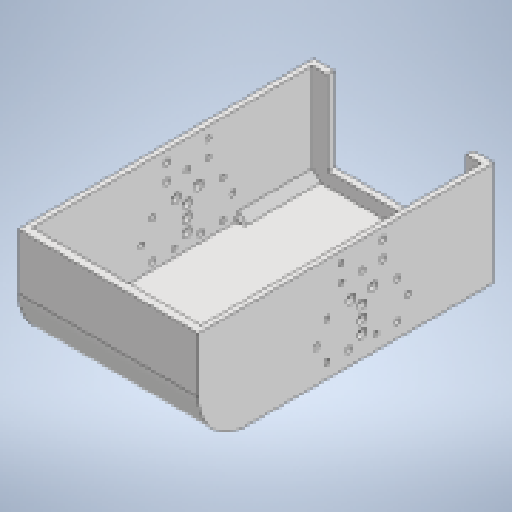
# Autodesk Inventor part: 车架
Saved by Autodesk Inventor 2025.1 (Build 291241000, 241)
## iProperties
Created: 2025-08-27
Part Number: 车架
Material: 常规
Document SubType Name: Modeling
Designer: Piw
Density: 1 g/cm^3
Appearance: 默认
Author: Piw
Autodesk Inventor part; units mm, degrees
ref_plane "YZ Plane" through (0, 0, 0) normal (1, 0, 0) x (0, 1, 0)
ref_plane "XZ Plane" through (0, 0, 0) normal (0, 1, 0) x (-1, 0, 0)
ref_plane "XY Plane" through (0, 0, 0) normal (0, 0, 1) x (1, 0, 0)
sketch "草图1" plane through (0, 0, 0) normal (0, 0, 1) x (1, 0, 0)
  line L0 (0, 5) -> (61, 5)
  line L1 (61, 5) -> (61, 75)
  line L2 (61, 75) -> (65, 75)
  line L3 (65, 75) -> (65, 0)
  line L4 (65, 0) -> (0, 0)
  line L5 (0, 34.2328) -> (0, -13.4923)
  line L6 (0, 5) -> (-61, 5)
  line L7 (-61, 5) -> (-61, 75)
  line L8 (-65, 75) -> (-65, 0)
  line L9 (-65, 0) -> (0, 0)
  line L10 (-61, 75) -> (-65, 75)
  dimension "d0" = 5
  dimension "d1" = 130
  dimension "d2" = 4
  dimension "d3" = 75
  constraints: 22 end point, 4 perpendicular, 4 symmetric about line, 2 vertical, 1 horizontal
  measures "d0" distance between parallel lines of L4 L0
  measures "d1" diameter of L3 L5
  measures "d2" distance between parallel lines of L3 L1
  measures "d3" distance between parallel lines of L4 L2
extrude "拉伸1" add sketch "草图1" along normal blind 138
sketch "草图2" plane through (65, 0, 0) normal (1, 0, 0) x (0, 0, -1)
  line L0 (-107.5, 24) -> (-72.5, 24) construction
  line L1 (0, 5) -> (-138, 5) projected
  circle A0 centre (-72.5, 24) radius 15.5 construction
  circle A1 centre (-107.5, 24) radius 15.5 construction
  circle A2 centre (-57, 24) radius 2.1
  circle A3 centre (-123, 24) radius 2.1
  line L2 (-138, 0) -> (-138, 75) projected
  circle A4 centre (-115.25, 10.5766) radius 2.1
  circle A5 centre (-99.75, 10.5766) radius 2.1
  circle A6 centre (-92, 24) radius 2.1
  circle A7 centre (-99.75, 37.4234) radius 2.1
  circle A8 centre (-115.25, 37.4234) radius 2.1
  circle A9 centre (-64.75, 37.4234) radius 2.1
  circle A10 centre (-80.25, 37.4234) radius 2.1
  circle A11 centre (-88, 24) radius 2.1
  circle A12 centre (-80.25, 10.5766) radius 2.1
  circle A13 centre (-64.75, 10.5766) radius 2.1
  point P0 (0, 0)
  dimension "d8" = 31
  dimension "d9" = 31
  dimension "d6" = 35
  dimension "d10" = 4.2
  dimension "d11" = 4.2
  dimension "d12" = 15
  dimension "d15" = 360
  dimension "d19" = 360
  dimension "d24" = 19
  constraints: 12 centre point, 2 coincident, 2 end point, 2 horizontal alignment, 2 point on line, 1 horizontal, 30 other
  measures "d6" distance of L0.start L0.end
  measures "d10" diameter of A2
  measures "d11" diameter of A3
  measures "d12" distance from line of L2 A3.centre
  measures "d24" distance between parallel lines of L1 L0
extrude "拉伸2" cut sketch "草图2" against normal blind 150 contours A2 | A3 | A4 | A5 | A8 | A9 | A12 | A13
sketch "草图3" plane through (65, 0, 0) normal (1, 0, 0) x (0, 0, -1)
  circle A0 centre (-90, 34) radius 3.25 projected
  circle A1 centre (-90, 25) radius 3.25 projected
  circle A2 centre (-90, 16) radius 3.25 projected
  circle A3 centre (-98, 41.2575) radius 3.25 projected
  circle A4 centre (-82, 41.2575) radius 3.25 projected
  point P0 (0, 0)
extrude "拉伸3" cut sketch "草图3" against normal blind 150
sketch "草图4" plane through (0, 0, 0) normal (0, 0, -1) x (-1, 0, 0)
  line L0 (-65, 0) -> (-65, 75) projected
  line L1 (65, 0) -> (-65, 0) projected
  line L2 (65, 75) -> (65, 0) projected
  line L3 (-65, 75) -> (-50, 75)
  line L4 (-50, 75) -> (-50, 15)
  line L5 (-50, 15) -> (50, 15)
  line L6 (50, 15) -> (50, 75)
  line L7 (50, 75) -> (65, 75)
  point P0 (0, 0)
  dimension "d27" = 15
  dimension "d28" = 15
  dimension "d29" = 15
  constraints: 10 end point, 4 perpendicular, 1 horizontal, 1 point on line
  measures "d27" distance between parallel lines of L1 L5
  measures "d28" distance between parallel lines of L2 L6
  measures "d29" distance between parallel lines of L4 L0
extrude "拉伸4" add sketch "草图4" along normal blind 5
sketch "草图5" plane through (0, 0, 0) normal (0, 0, 1) x (1, 0, 0)
  line L0 (61, 75) -> (61, 5) projected
  line L1 (50, 75) -> (61, 75) projected
  line L2 (50, 15) -> (50, 75) projected
  line L3 (-50, 15) -> (50, 15) projected
  line L4 (-50, 75) -> (-50, 15) projected
  line L5 (-61, 75) -> (-50, 75) projected
  line L6 (-61, 5) -> (-61, 75) projected
  line L7 (61, 5) -> (-61, 5) projected
  line L8 (61, 11) -> (55, 5)
  line L9 (0, 97.2027) -> (0, -45.2903)
  line L10 (-61, 11) -> (-55, 5)
  point P0 (0, 0)
  dimension "d32" = 45
  dimension "d33" = 6
  constraints: 6 end point, 2 point on line, 2 symmetric about line, 2 vertical
  measures "d32" angle of L0 L8
  measures "d33" horizontal distance of L8.end L8.start
extrude "拉伸5" add sketch "草图5" along normal blind 55 contours L0 L7 L8 | L7 L6 L10
chamfer "倒角1" distance 2 angle 45 2 edges at (58, 8, 55) (-58, 8, 55)
sketch "草图7" plane through (0, 0, 138) normal (0, 0, 1) x (1, 0, 0)
  line L0 (-65, 0) -> (65, 0) projected
  line L1 (65, 0) -> (65, 75) projected
  line L2 (65, 75) -> (61, 75) projected
  line L3 (61, 75) -> (61, 5) projected
  line L4 (61, 5) -> (-61, 5) projected
  line L5 (-61, 5) -> (-61, 75) projected
  line L6 (-61, 75) -> (-65, 75) projected
  line L7 (-65, 75) -> (-65, 0) projected
  point P0 (0, 0)
extrude "拉伸6" add sketch "草图7" along normal blind 25
sketch "草图13" plane through (-65, 0, -5) normal (-1, 0, 0) x (0, 0, 1)
  line L0 (80, 55) -> (110, 55) construction
  line L1 (110, 55) -> (110, 67) construction
  line L2 (110, 67) -> (80, 67) construction
  line L3 (80, 67) -> (80, 55) construction
  line L4 (80, 55) -> (110, 67) construction
  line L5 (110, 55) -> (80, 67) construction
  line L6 (0, 75) -> (168, 75) projected
  circle A0 centre (95, 34) radius 3.25 projected
  line L7 (95, 34) -> (95, 46.2012) construction
  circle A1 centre (80, 55) radius 2.1
  circle A2 centre (110, 55) radius 2.1
  circle A3 centre (95, 55) radius 2.1
  circle A4 centre (80, 67) radius 2.1
  circle A5 centre (110, 67) radius 2.1
  point P0 (5, 0)
  point P1 (95, 61)
  point P2 (233, 75)
  dimension "d62" = 8
  dimension "d63" = 30
  dimension "d64" = 20
  dimension "d65" = 4.2
  dimension "d66" = 4.2
  dimension "d67" = 4.2
  dimension "d68" = 4.2
  dimension "d69" = 4.2
  constraints: 14 end point, 5 centre point, 4 coincident, 3 midpoint, 2 parallel, 1 horizontal, 1 perpendicular, 1 point on line, 1 vertical
  measures "d62" distance between parallel lines of L6 L2
  measures "d63" distance between parallel lines of L1 L3
  measures "d64" distance between parallel lines of L6 L0
  measures "d65" diameter of A1
  measures "d66" diameter of A2
  measures "d67" diameter of A3
  measures "d68" diameter of A4
  measures "d69" diameter of A5
extrude "拉伸11" cut sketch "草图13" against normal blind 150 contours A1 | A2 | A3 | A4 | A5
sketch "草图14" plane through (0, 0, 163) normal (0, 0, 1) x (1, 0, 0)
  line L0 (65, 0) -> (65, 75) projected
  line L1 (65, 75) -> (61, 75) projected
  line L2 (61, 75) -> (61, 5) projected
  line L3 (61, 5) -> (-61, 5) projected
  line L4 (-61, 5) -> (-61, 75) projected
  line L5 (-61, 75) -> (-65, 75) projected
  line L6 (-65, 75) -> (-65, 0) projected
  line L7 (-65, 0) -> (65, 0) projected
  point P0 (0, 0)
extrude "拉伸12" add sketch "草图14" along normal blind 45
sketch "草图15" plane through (-55, 5, 0) normal (0, 1, 0) x (1, 0, 0)
  line L0 (-6, -55) -> (-6, -208) projected
  line L1 (116, 0) -> (116, -208) projected
  line L2 (-6, -208) -> (116, -208)
  line L3 (116, -208) -> (116, -202)
  line L4 (116, -202) -> (-6, -202)
  line L5 (-6, -202) -> (-6, -208)
  point P0 (55, 0)
  point P1 (-6, -202)
  dimension "d74" = 6
  constraints: 8 end point, 2 parallel, 1 horizontal, 1 perpendicular, 1 point on line
  measures "d74" distance between parallel lines of L2 L4
extrude "拉伸13" add sketch "草图15" along normal up to surface (70 mm away)
fillet "圆角2" radius 30 1 edges at (0, 5, 202)
fillet "圆角3" radius 35 1 edges at (0, 0, 208)
